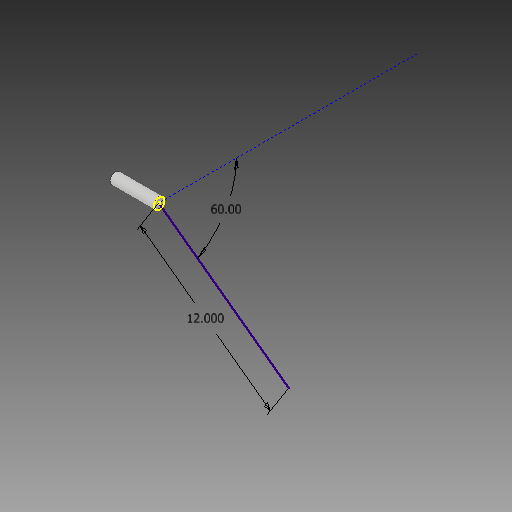
# Autodesk Inventor part: Sling
Saved by Autodesk Inventor 2019 (Build 230136000, 136)
## iProperties
Created: 2019-07-23
Part Number: Sling
Material: Generic
Document SubType Name: Modeling
Designer: AlphaGoldOmegaSilver
Density: 1 g/cm^3
Appearance: Default
Mass: 6.43518 g
Surface Area: 22.8018 cm^2
Volume: 6.43518 cm^3
Author: AlphaGoldOmegaSilver
Autodesk Inventor part; units mm, degrees
ref_plane "YZ Plane" through (0, 0, 0) normal (1, 0, 0) x (0, 1, 0)
ref_plane "XZ Plane" through (0, 0, 0) normal (0, 1, 0) x (-1, 0, 0)
ref_plane "XY Plane" through (0, 0, 0) normal (0, 0, 1) x (1, 0, 0)
sketch "Sketch1" plane through (0, 0, 0) normal (1, 0, 0) x (0, 1, 0)
  circle A0 centre (0, 0) radius 6.35
  dimension "d0" = 12.7
  constraints: 1 centre point, 1 coincident
  measures "d0" diameter of A0
extrude "Extrusion1" add sketch "Sketch1" along normal blind 50.8
sketch "Sketch2" plane through (50.8, 0, 0) normal (1, 0, 0) x (0, 0, -1)
  circle A0 centre (0, 0) radius 6.35 projected
  line L0 (0, 0) -> (152.4, -263.9645)
  line L1 (0, 0) -> (304.8, 0) construction
  dimension "d3" = 304.8
  dimension "d4" = 60
  constraints: 4 end point, 1 equal length, 1 horizontal
  measures "d3" distance of L0.start L0.end
  measures "d4" angle of L0 L1
body "Solid1"
